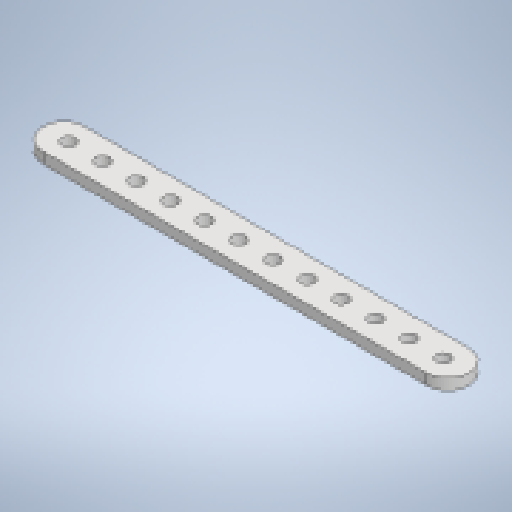
# Autodesk Inventor part: anchor-point
Saved by Autodesk Inventor 2024.1 (Build 281209000, 209)
## iProperties
Created: 2025-06-08
Part Number: anchor-point
Material: Generic
Document SubType Name: Modeling
Designer: iwheard
Density: 1 g/cm^3
Appearance: Default
Author: iwheard
Autodesk Inventor part; units mm, degrees
ref_plane "YZ Plane" through (0, 0, 0) normal (1, 0, 0) x (0, 1, 0)
ref_plane "XZ Plane" through (0, 0, 0) normal (0, 1, 0) x (-1, 0, 0)
ref_plane "XY Plane" through (0, 0, 0) normal (0, 0, 1) x (1, 0, 0)
sketch "Sketch1" plane through (0, 0, 0) normal (0, 1, 0) x (-1, 0, 0)
  line L0 (-50, 0) -> (50, 0)
  line L1 (50, 0) -> (50, 10)
  line L2 (50, 10) -> (-50, 10)
  line L3 (-50, 10) -> (-50, 0)
  point P0 (0, 0)
  dimension "d0" = 10
  dimension "d1" = 100
  dimension "d2" = 50
  constraints: 8 end point, 2 parallel, 1 horizontal, 1 horizontal alignment, 1 perpendicular
  measures "d0" distance between parallel lines of L2 L0
  measures "d1" distance between parallel lines of L1 L3
  measures "d2" distance from line of L1 point (0, 0)
extrude "Extrusion1" add sketch "Sketch1" along normal blind 2.5
sketch "Sketch2" plane through (0, 2.5, 0) normal (0, 1, 0) x (1, 0, 0)
  circle A0 centre (44, -5) radius 1.6
  line L0 (50, -10) -> (50, 0) projected
  line L1 (-50, -10) -> (50, -10) projected
  line L2 (50, 0) -> (-50, 0) projected
  line L3 (-50, 0) -> (-50, -10) projected
  circle A1 centre (36, -5) radius 1.6
  circle A2 centre (28, -5) radius 1.6
  circle A3 centre (20, -5) radius 1.6
  circle A4 centre (12, -5) radius 1.6
  circle A5 centre (4, -5) radius 1.6
  circle A6 centre (-4, -5) radius 1.6
  circle A7 centre (-12, -5) radius 1.6
  circle A8 centre (-20, -5) radius 1.6
  circle A9 centre (-28, -5) radius 1.6
  circle A10 centre (-36, -5) radius 1.6
  circle A11 centre (-44, -5) radius 1.6
  point P0 (0, 0)
  dimension "d5" = 6
  dimension "d6" = 3.2
  dimension "d7" = 10
  dimension "d8" = 5
  dimension "d10" = 100
  dimension "d13" = 8
  dimension "d18" = 6
  constraints: 12 centre point, 1 horizontal, 22 other
  measures "d5" distance from line of A0.centre L0
  measures "d6" diameter of A0
  measures "d7" distance between parallel lines of L1 L2
  measures "d8" distance from line of L2 A0.centre
  measures "d10" distance between parallel lines of L3 L0
  measures "d13" distance of A0.centre A1.centre
  measures "d18" distance from line of L3 A11.centre
extrude "Extrusion2" cut sketch "Sketch2" against normal through all contours A0 | A1 | A2 | A3 | A4 | A5 | A6 | A7 | A8 | A9 | A10 | A11
fillet "Fillet1" radius 5 4 edges at (50, 1.25, 10) (50, 1.25, 0) (-50, 1.25, 10) (-50, 1.25, 0)
equation "\"d2\" = 0.5 * d1"
equation "\"d8\" = 0.5 * d7"
body "Solid1"
